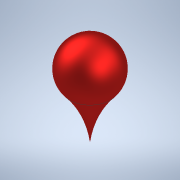
# Autodesk Inventor part: Marker
Saved by Autodesk Inventor 2021 (Build 250183000, 183)
## iProperties
Created: 2020-04-19
Part Number: Marker
Material: Generic
Document SubType Name: Modeling
Designer: bapel
Density: 1 g/cm^3
Appearance: Default
Author: bapel
Autodesk Inventor part; units mm, degrees
ref_plane "YZ Plane" through (0, 0, 0) normal (1, 0, 0) x (0, 1, 0)
ref_plane "XZ Plane" through (0, 0, 0) normal (0, 1, 0) x (-1, 0, 0)
ref_plane "XY Plane" through (0, 0, 0) normal (0, 0, 1) x (1, 0, 0)
sketch "Sketch1" plane through (0, 0, 0) normal (0, 1, 0) x (-1, 0, 0)
  circle A0 centre (0, 0) radius 12.7
  line L0 (0, 12.7) -> (0, -12.7)
  dimension "d0" = 25.4
  constraints: 2 end point, 2 point on circle, 1 centre point, 1 coincident, 1 vertical
  measures "d0" diameter of A0
revolve "Revolution1" add sketch "Sketch1" angle 360 about axis through (0, 0, 12.7) along (0, 0, -1) picked at (2.6394, 3.3098) contours A0 L0
sketch "Sketch2" plane through (0, 0, 0) normal (0, 0, 1) x (1, 0, 0)
  circle A0 centre (0, 0) radius 12.7 projected
  arc A1 (0, -30.3622) -> (-9.7611, -8.1247) centre (-42.4069, -35.7156) ccw
  line L0 (0, -30.3622) -> (0, 0)
  point P0 (0, -12.7)
  point P1 (-9.6663, -8.2373)
  constraints: 2 end point, 2 point on circle, 1 centre point, 1 vertical, 2 other
revolve "Revolution2" add sketch "Sketch2" angle 360 about axis through (0, -30.3622, 0) along (0, 1, 0) contours A0 L0 A1
body "Solid1"
